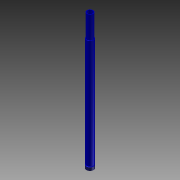
# Autodesk Inventor part: 13_0204_023
Saved by Autodesk Inventor 2012 SP1 (Build 160190100, 190)
## iProperties
Created: 2013-04-03
Part Number: 13_0204_023
Material: Default
Document SubType Name: Modeling
Designer: vogel
Density: 1 g/cm^3
Author: vogel
Autodesk Inventor part; units mm, degrees
ref_plane "YZ Plane" through (0, 0, 0) normal (1, 0, 0) x (0, 1, 0)
ref_plane "XZ Plane" through (0, 0, 0) normal (0, 1, 0) x (-1, 0, 0)
ref_plane "XY Plane" through (0, 0, 0) normal (0, 0, 1) x (1, 0, 0)
sketch "Skizze1" plane through (0, 0, 0) normal (0, 0, 1) x (1, 0, 0)
  circle A0 centre (0, 0) radius 8
  circle A1 centre (0, 0) radius 6
  dimension "d0" = 2
  dimension "d1" = 16
  constraints: 2 centre point, 2 coincident
  measures "d0" radial gap between concentric circles of A0 A1
  measures "d1" diameter of A0
extrude "Extrusion1" add sketch "Skizze1" along normal blind 298
sketch "Skizze2" plane through (0, 0, 298) normal (0, 0, 1) x (1, 0, 0)
  circle A0 centre (0, 0) radius 8 projected
  circle A1 centre (0, 0) radius 7
  dimension "d4" = 14
  constraints: 1 centre point, 1 coincident
  measures "d4" diameter of A1
extrude "Extrusion2" cut sketch "Skizze2" against normal blind 50
sketch "Skizze3" plane through (0, 0, 248) normal (0, 0, 1) x (1, 0, 0)
  circle A0 centre (0, 0) radius 8 projected
  circle A1 centre (0, 0) radius 7.75
  dimension "d7" = 15.5
  constraints: 1 centre point, 1 coincident
  measures "d7" diameter of A1
extrude "Extrusion3" cut sketch "Skizze3" against normal through all
sketch "Skizze4" plane through (0, 0, 0) normal (0, 0, -1) x (-1, 0, 0)
  circle A0 centre (0, 0) radius 7.75 projected
  circle A1 centre (0, 0) radius 6 projected
  circle A2 centre (0, 0) radius 8
  dimension "d10" = 16
  constraints: 1 centre point, 1 coincident
  measures "d10" diameter of A2
extrude "Extrusion4" add sketch "Skizze4" against normal blind 9 contours A2
sketch "Skizze5" plane through (0, 0, 0) normal (0, 1, 0) x (-1, 0, 0)
  line L0 (-8, 9) -> (8, 9) projected
  line L1 (8, 0) -> (-8, 0) projected
  line L2 (8, 0) -> (8, 9) projected
  line L3 (6, 0) -> (6, 298) projected
  line L4 (7.75, 248) -> (7.75, 9) projected
  line L5 (0, -50) -> (0, 300) projected
  line L6 (8, 7.5) -> (7.25, 7.5)
  line L7 (7.25, 7.5) -> (7.25, 9)
  line L8 (8, 9) -> (7.25, 9)
  line L9 (8, 9) -> (8, 7.5)
  point P0 (0, 0)
  dimension "d17" = 1.5
  dimension "d18" = 14.5
  constraints: 8 end point, 2 collinear, 2 point on line, 1 parallel, 1 perpendicular
  measures "d17" distance of L2.end L6.start
  measures "d18" diameter of L7 L5
revolve "Umdrehung1" cut sketch "Skizze5" angle 360 about axis through (0, 0, -10) along (0, 0, 1) contours L0 L2 L6 L7
chamfer "Fase1" distance 0.75 angle 45 1 edges at (8, 0, 7.5)
thread "Gewinde3" size "M16x1" class "6g" standard "ANSI Metric M Profile" full length
fillet "Rundung1" radius 0.5 1 edges at (-7, 0, 248)
